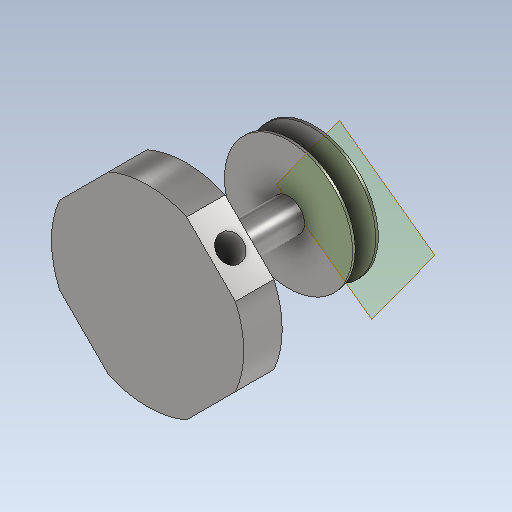
# Autodesk Inventor part: shaft
Saved by Autodesk Inventor 2021 (Build 250183000, 183)
## iProperties
Created: 2021-06-18
Part Number: shaft
Material: Stal, stopowa
Document SubType Name: Modeling
Designer: Wojciech Wołczek
Density: 7.73 g/cm^3
Appearance: Częściowo polerowana
Author: Wojciech Wołczek
Autodesk Inventor part; units mm, degrees
ref_plane "YZ Plane" through (0, 0, 0) normal (1, 0, 0) x (0, 1, 0)
ref_plane "XZ Plane" through (0, 0, 0) normal (0, 1, 0) x (-1, 0, 0)
ref_plane "XY Plane" through (0, 0, 0) normal (0, 0, 1) x (1, 0, 0)
ref_plane "Płaszczyzna konstrukcyjna1" through (120.7768, 82.8896, 9.246) normal (0, 0, -1) x (-0.5875457, -0.809191, 0)
sketch "Szkic1" plane through (120.7768, 82.8896, 9.246) normal (0, 0, -1) x (-0.5875457, -0.809191, 0)
  circle A0 centre (18.3881, 39.1184) radius 12.5
  circle A1 centre (66.5199, 68.1563) radius 12.5 projected
  point P0 (138.0354, 49.03)
  dimension "d0" = 25
  constraints: 1 centre point
  measures "d0" diameter of A0
extrude "Wyciągnięcie proste1" add sketch "Szkic1" along normal blind 20 and the other way blind 110 contours A1
sketch "Szkic2" plane through (120.7768, 82.8896, 9.246) normal (0, 0, -1) x (-0.5875457, -0.809191, 0)
  circle A0 centre (66.5199, 68.1563) radius 12.5 projected
  circle A1 centre (66.5199, 68.1563) radius 50
  point P0 (138.0354, 49.03)
  dimension "d5" = 100
  constraints: 1 centre point, 1 coincident
  measures "d5" diameter of A1
extrude "Wyciągnięcie proste2" add sketch "Szkic2" along normal blind 10
chamfer "Faza1" distance 37 distance2 8 1 edges at (55.9191, 109.5667, -0.754) measured on face at (55.6253, 109.1621, -0.754)
sketch "Szkic3" plane through (26.5418, 69.1072, -10.754) normal (0, 0, -1) x (-1, 0, 0)
  circle A0 centre (0, 0) radius 50
  point P0 (26.5418, -69.1072)
  dimension "d11" = 100
  constraints: 1 centre point
  measures "d11" diameter of A0
extrude "Wyciągnięcie proste3" add sketch "Szkic3" against normal blind 10
chamfer "Faza2" distance 37 distance2 8 1 edges at (76.5418, 69.1072, -0.754) measured on face at (76.0418, 69.1072, -0.754)
sketch "Szkic4" plane through (26.5418, 69.1072, 119.246) normal (0, 0, 1) x (1, 0, 0)
  circle A0 centre (0, 0) radius 75
  point P0 (-26.5418, -69.1072)
  dimension "d17" = 150
  constraints: 1 centre point
  measures "d17" diameter of A0
extrude "Wyciągnięcie proste4" add sketch "Szkic4" against normal blind 30
sketch "Szkic5" plane through (26.5418, 69.1072, 119.246) normal (0, 0, 1) x (1, 0, 0)
  line L0 (0, 98.9949) -> (98.9949, 0)
  line L1 (98.9949, 0) -> (0, -98.9949)
  line L2 (0, -98.9949) -> (-98.9949, 0)
  line L3 (-98.9949, 0) -> (0, 98.9949)
  line L4 (0, 98.9949) -> (0, -98.9949) construction
  line L5 (98.9949, 0) -> (-98.9949, 0) construction
  line L6 (0, 98.9949) -> (140, 98.9949) construction
  circle A0 centre (0, 0) radius 12.5 projected
  circle A1 centre (0, 0) radius 75
  point P0 (-26.5418, -69.1072)
  point P1 (-68.5369, -30.458)
  point P2 (-30.458, -68.5369)
  point P3 (-30.458, 68.5369)
  point P4 (-68.5369, 30.458)
  point P5 (68.5369, 30.458)
  point P6 (30.458, 68.5369)
  point P7 (30.458, -68.5369)
  point P8 (68.5369, -30.458)
  dimension "d20" = 140
  dimension "d21" = 45
  dimension "d22" = 140
  dimension "d23" = 150
  constraints: 14 end point, 2 midpoint, 2 parallel, 1 centre point, 1 coincident, 1 equal length, 1 horizontal, 1 perpendicular
  measures "d20" distance of L0.start L0.end
  measures "d21" angle of L0 L6
  measures "d22" distance of L0.end L1.end
  measures "d23" diameter of A1
extrude "Wyciągnięcie proste5" cut sketch "Szkic5" against normal blind 30 contours A1 L0 | L3 A1 | L2 A1 | A1 L1
sketch "Szkic6" plane through (56.9998, 0.5703, 89.246) normal (0.7071068, -0.7071068, 0) x (0.7071068, 0.7071068, 0)
  circle A0 centre (27.509, 15) radius 10
  point P0 (-40.7082, -89.246)
  dimension "d26" = 20
  constraints: 1 centre point
  measures "d26" diameter of A0
extrude "Wyciągnięcie proste6" cut sketch "Szkic6" against normal through all
sketch "Szkic7" plane through (95.0787, 99.5652, 119.246) normal (0.7071068, 0.7071068, 0) x (0.7071068, -0.7071068, 0)
  line L0 (0, 0) -> (-53.8516, 0) projected
  line L1 (0, 30) -> (0, 0) projected
  line L2 (-53.8516, 30) -> (0, 30) projected
  line L3 (-53.8516, 0) -> (-53.8516, 30) projected
  circle A0 centre (-26.9258, 15) radius 10
  point P0 (3.1724, 119.246)
  dimension "d29" = 20
  constraints: 1 centre point
  measures "d29" diameter of A0
extrude "Wyciągnięcie proste7" cut sketch "Szkic7" against normal through all contours A0
